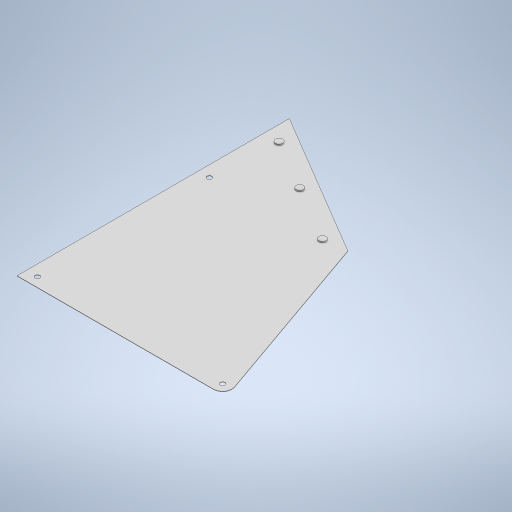
# Autodesk Inventor part: base_main_pcb_p2_itr3
Saved by Autodesk Inventor 2024 (Build 280153000, 153)
## iProperties
Created: 2026-03-21
Part Number: base_main_pcb_p2_itr3
Material: Generic
Document SubType Name: Modeling
Designer: schar
Density: 1 g/cm^3
Appearance: Default
Author: schar
Autodesk Inventor part; units mm, degrees
ref_plane "YZ Plane" through (0, 0, 0) normal (1, 0, 0) x (0, 1, 0)
ref_plane "Work Plane1" through (-205, 2.4, 12.8522) normal (0, 1, 0) x (1, 0, 0)
sketch "Sketch1" plane through (-205, 2.4, 12.8522) normal (0, 1, 0) x (1, 0, 0)
  line L0 (138.3655, -268.878) -> (91, -133.6728) projected
  line L1 (97.1039, -151.0965) -> (0, -93.5034)
  line L2 (0, 0) -> (0, -277.1478) projected
  circle A0 centre (132.5, -270.9328) radius 1.675 projected
  circle A1 centre (132.5, -270.9328) radius 6.215
  line L3 (138.3655, -268.878) -> (97.1039, -151.0965)
  line L4 (132.5, -277.1478) -> (0, -277.1478)
  line L5 (0, -277.1478) -> (0, -93.5034)
  circle A2 centre (82.1326, -153.2062) radius 2.5 projected
  circle A3 centre (82.1326, -153.2062) radius 2.5
  circle A4 centre (44.6303, -131.0762) radius 2.5 projected
  circle A5 centre (44.6303, -131.0762) radius 2.5
  circle A6 centre (10.5733, -110.9794) radius 2.5 projected
  circle A7 centre (10.5733, -110.9794) radius 2.5
  circle A8 centre (7.5, -154.9228) radius 1.675 projected
  circle A9 centre (7.5, -154.9228) radius 1.675
  circle A10 centre (7.5, -270.9328) radius 1.675
  point P0 (205, 12.8522)
  constraints: 8 end point, 6 centre point, 5 coincident, 2 point on circle, 2 point on line, 1 collinear, 1 horizontal
extrude "Extrusion1" add sketch "Sketch1" along normal blind 0.2
ref_plane "Work Plane2" through (-205, 2.4, 12.8522) normal (0, 1, 0) x (1, 0, 0)
sketch "Sketch2" plane through (-205, 2.4, 12.8522) normal (0, 1, 0) x (1, 0, 0)
  circle A0 centre (82.1326, -153.2062) radius 2.5 projected
  circle A1 centre (82.1326, -153.2062) radius 2.5
  circle A2 centre (44.6303, -131.0762) radius 2.5 projected
  circle A3 centre (44.6303, -131.0762) radius 2.5
  circle A4 centre (10.5733, -110.9794) radius 2.5 projected
  circle A5 centre (10.5733, -110.9794) radius 2.5
  point P0 (205, 12.8522)
  constraints: 3 centre point, 3 coincident
extrude "Extrusion2" add sketch "Sketch2" along normal blind 1
body "Solid2"
